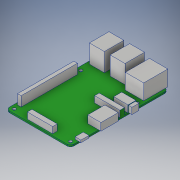
# Autodesk Inventor part: RaspberryPi3B+
Saved by Autodesk Inventor 2017 (Build 210142000, 142)
## iProperties
Created: 2018-08-04
Part Number: RaspberryPi3B+
Material: Aluminum 6061
Document SubType Name: Modeling
Designer: Jake
Density: 2.7 g/cm^3
Appearance: Aluminum - Flat
Author: Jake
Autodesk Inventor part; units mm, degrees
ref_plane "YZ Plane" through (0, 0, 0) normal (1, 0, 0) x (0, 1, 0)
ref_plane "XZ Plane" through (0, 0, 0) normal (0, 1, 0) x (-1, 0, 0)
ref_plane "XY Plane" through (0, 0, 0) normal (0, 0, 1) x (1, 0, 0)
sketch "Sketch1" plane through (0, 0, 0) normal (0, 1, 0) x (-1, 0, 0)
  line L0 (28, 42.5) -> (-28, 42.5)
  line L1 (-28, 42.5) -> (-28, -42.5)
  line L2 (-28, -42.5) -> (28, -42.5)
  line L3 (28, -42.5) -> (28, 42.5)
  point P0 (0, 0)
  point P1 (28, 0)
  point P2 (0, -42.5)
  dimension "d0" = 85
  dimension "d1" = 56
  constraints: 8 end point, 2 midpoint, 2 parallel, 1 horizontal, 1 horizontal alignment, 1 perpendicular, 1 vertical alignment
  measures "d0" distance of L2.end L0.start
  measures "d1" distance of L1.end L2.end
extrude "Extrusion1" add sketch "Sketch1" along normal blind 1.43
sketch "Sketch2" plane through (0, 1.43, 0) normal (0, 1, 0) x (1, 0, 0)
  line L0 (-28, -42.5) -> (28, -42.5) projected
  line L1 (28, -42.5) -> (28, 42.5) projected
  line L2 (28, 42.5) -> (-28, 42.5) projected
  line L3 (-28, 42.5) -> (-28, -42.5) projected
  circle A0 centre (-24.5, -39) radius 1.375
  circle A1 centre (-24.5, 19) radius 1.375
  circle A2 centre (24.5, 19) radius 1.375
  circle A3 centre (24.5, -39) radius 1.375
  point P0 (0, 0)
  dimension "d4" = 2.75
  dimension "d5" = 2.75
  dimension "d6" = 2.75
  dimension "d7" = 2.75
  dimension "d8" = 49
  dimension "d9" = 58
  dimension "d10" = 3.5
  dimension "d11" = 3.5
  constraints: 4 centre point, 2 horizontal alignment, 2 vertical alignment
  measures "d4" diameter of A0
  measures "d5" diameter of A1
  measures "d6" diameter of A2
  measures "d7" diameter of A3
  measures "d8" distance of A3.centre A0.centre
  measures "d9" distance of A1.centre A0.centre
  measures "d10" distance from line of A3.centre L0
  measures "d11" distance from line of L3 A0.centre
extrude "Extrusion2" cut sketch "Sketch2" against normal through all contours A0 | A1 | A2 | A3
fillet "Fillet1" radius 3 4 edges at (-28, 0.715, 42.5) (28, 0.715, 42.5) (28, 0.715, -42.5) (-28, 0.715, -42.5)
sketch "Sketch3" plane through (0, 1.43, 0) normal (0, 1, 0) x (1, 0, 0)
  circle A0 centre (24.5, 19) radius 1.375 projected
  circle A1 centre (-24.5, -39) radius 1.375 projected
  circle A2 centre (-24.5, 19) radius 1.375 projected
  circle A3 centre (24.5, -39) radius 1.375 projected
  arc A4 (-25, 42.5) -> (-28, 39.5) centre (-25, 39.5) ccw projected
  line L0 (-28, 39.5) -> (-28, -39.5) projected
  arc A5 (-28, -39.5) -> (-25, -42.5) centre (-25, -39.5) ccw projected
  line L1 (-25, -42.5) -> (25, -42.5) projected
  arc A6 (25, -42.5) -> (28, -39.5) centre (25, -39.5) ccw projected
  line L2 (28, -39.5) -> (28, 39.5) projected
  arc A7 (28, 39.5) -> (25, 42.5) centre (25, 39.5) ccw projected
  line L3 (25, 42.5) -> (-25, 42.5) projected
  line L4 (-25.5, 27.5) -> (-12.5, 27.5)
  line L5 (-12.5, 27.5) -> (-12.5, 44.5)
  line L6 (-12.5, 44.5) -> (-25.5, 44.5)
  line L7 (-25.5, 44.5) -> (-25.5, 27.5)
  line L8 (-7.5, 27.5) -> (5.5, 27.5)
  line L9 (5.5, 27.5) -> (5.5, 44.5)
  line L10 (5.5, 44.5) -> (-7.5, 44.5)
  line L11 (-7.5, 44.5) -> (-7.5, 27.5)
  point P0 (0, 0)
  point P1 (-19, 44.5)
  point P2 (-1, 44.5)
  dimension "d15" = 2
  dimension "d16" = 29
  dimension "d17" = 47
  dimension "d18" = 13
  dimension "d19" = 13
  dimension "d20" = 17
  constraints: 16 end point, 4 parallel, 2 horizontal, 2 midpoint, 2 perpendicular, 2 point on line
  measures "d15" distance between parallel lines of L6 L3
  measures "d16" distance from line of point (-1, 44.5) L2
  measures "d17" distance from line of point (-19, 44.5) L2
  measures "d18" distance of L5.end L6.end
  measures "d19" distance of L9.end L10.end
  measures "d20" distance of L6.end L4.start
extrude "Extrusion3" add sketch "Sketch3" along normal blind 16 contours L3 L5 L4 L7 A4 | A4 L7 L6 L5 L3 | L11 L10 L9 L3 | L3 L9 L8 L11
sketch "Sketch4" plane through (0, 1.43, 0) normal (0, 1, 0) x (1, 0, 0)
  line L0 (-7.5, 27.5) -> (-7.5, 42.5) projected
  line L1 (-7.5, 42.5) -> (-12.5, 42.5) projected
  line L2 (-12.5, 42.5) -> (-12.5, 27.5) projected
  line L3 (-12.5, 27.5) -> (-25.5, 27.5) projected
  line L4 (-25.5, 27.5) -> (-25.5, 42.458) projected
  arc A0 (-25.5, 42.458) -> (-28, 39.5) centre (-25, 39.5) ccw projected
  line L5 (-28, 39.5) -> (-28, -39.5) projected
  arc A1 (-28, -39.5) -> (-25, -42.5) centre (-25, -39.5) ccw projected
  line L6 (-25, -42.5) -> (25, -42.5) projected
  arc A2 (25, -42.5) -> (28, -39.5) centre (25, -39.5) ccw projected
  line L7 (28, -39.5) -> (28, 39.5) projected
  arc A3 (28, 39.5) -> (25, 42.5) centre (25, 39.5) ccw projected
  line L8 (25, 42.5) -> (5.5, 42.5) projected
  line L9 (5.5, 42.5) -> (5.5, 27.5) projected
  line L10 (5.5, 27.5) -> (-7.5, 27.5) projected
  circle A4 centre (24.5, 19) radius 1.375 projected
  circle A5 centre (-24.5, -39) radius 1.375 projected
  circle A6 centre (-24.5, 19) radius 1.375 projected
  circle A7 centre (24.5, -39) radius 1.375 projected
  line L11 (-7.5, 27.5) -> (5.5, 27.5) projected
  line L12 (5.5, 27.5) -> (5.5, 44.5) projected
  line L13 (5.5, 44.5) -> (-7.5, 44.5) projected
  line L14 (-7.5, 44.5) -> (-7.5, 27.5) projected
  line L15 (9.75, 23.5) -> (25.75, 23.5)
  line L16 (25.75, 23.5) -> (25.75, 44.5)
  line L17 (25.75, 44.5) -> (9.75, 44.5)
  line L18 (9.75, 44.5) -> (9.75, 23.5)
  point P0 (0, 0)
  point P1 (17.75, 44.5)
  dimension "d23" = 10.25
  dimension "d24" = 21
  dimension "d25" = 16
  constraints: 8 end point, 2 parallel, 1 collinear, 1 horizontal, 1 midpoint, 1 perpendicular
  measures "d23" distance from line of point (17.75, 44.5) L7
  measures "d24" distance of L17.end L15.start
  measures "d25" distance of L16.end L17.end
extrude "Extrusion4" add sketch "Sketch4" along normal blind 13.5 contours L18 L17 L16 A3 L8 | L8 A3 L16 L15 L18
sketch "Sketch5" plane through (0, 1.43, 0) normal (0, 1, 0) x (1, 0, 0)
  line L0 (9.75, 23.5) -> (9.75, 42.5) projected
  line L1 (9.75, 42.5) -> (5.5, 42.5) projected
  line L2 (5.5, 42.5) -> (5.5, 27.5) projected
  line L3 (5.5, 27.5) -> (-7.5, 27.5) projected
  line L4 (-7.5, 27.5) -> (-7.5, 42.5) projected
  line L5 (-7.5, 42.5) -> (-12.5, 42.5) projected
  line L6 (-12.5, 42.5) -> (-12.5, 27.5) projected
  line L7 (-12.5, 27.5) -> (-25.5, 27.5) projected
  line L8 (-25.5, 27.5) -> (-25.5, 42.458) projected
  arc A0 (-25.5, 42.458) -> (-28, 39.5) centre (-25, 39.5) ccw projected
  line L9 (-28, 39.5) -> (-28, -39.5) projected
  arc A1 (-28, -39.5) -> (-25, -42.5) centre (-25, -39.5) ccw projected
  line L10 (-25, -42.5) -> (25, -42.5) projected
  arc A2 (25, -42.5) -> (28, -39.5) centre (25, -39.5) ccw projected
  line L11 (28, -39.5) -> (28, 39.5) projected
  arc A3 (28, 39.5) -> (25.75, 42.4047) centre (25, 39.5) ccw projected
  line L12 (25.75, 42.4047) -> (25.75, 23.5) projected
  line L13 (25.75, 23.5) -> (9.75, 23.5) projected
  circle A4 centre (24.5, 19) radius 1.375 projected
  circle A5 centre (-24.5, -39) radius 1.375 projected
  circle A6 centre (-24.5, 19) radius 1.375 projected
  circle A7 centre (24.5, -39) radius 1.375 projected
  line L14 (-26.075, -34.5) -> (-22.925, -34.5)
  line L15 (-22.925, -34.5) -> (-22.925, 14.5)
  line L16 (-22.925, 14.5) -> (-26.075, 14.5)
  line L17 (-26.075, 14.5) -> (-26.075, -34.5)
  point P0 (0, 0)
  point P1 (-26.075, -10)
  point P2 (-24.5, -34.5)
  dimension "d28" = 3.15
  dimension "d29" = 49
  dimension "d31" = 29
  constraints: 8 end point, 2 midpoint, 2 parallel, 1 horizontal, 1 perpendicular, 1 vertical alignment
  measures "d28" distance of L15.end L16.end
  measures "d29" distance of L16.end L14.start
  measures "d31" vertical distance of point (-26.075, -10) A5.centre
extrude "Extrusion5" add sketch "Sketch5" along normal blind 8.5 contours L17 L16 L15 L14
sketch "Sketch6" plane through (0, 1.43, 0) normal (0, 1, 0) x (1, 0, 0)
  line L0 (-26.075, -34.5) -> (-26.075, 14.5) projected
  line L1 (-26.075, 14.5) -> (-22.925, 14.5) projected
  line L2 (-22.925, 14.5) -> (-22.925, -34.5) projected
  line L3 (-22.925, -34.5) -> (-26.075, -34.5) projected
  line L4 (9.75, 23.5) -> (9.75, 42.5) projected
  line L5 (9.75, 42.5) -> (5.5, 42.5) projected
  line L6 (5.5, 42.5) -> (5.5, 27.5) projected
  line L7 (5.5, 27.5) -> (-7.5, 27.5) projected
  line L8 (-7.5, 27.5) -> (-7.5, 42.5) projected
  line L9 (-7.5, 42.5) -> (-12.5, 42.5) projected
  line L10 (-12.5, 42.5) -> (-12.5, 27.5) projected
  line L11 (-12.5, 27.5) -> (-25.5, 27.5) projected
  line L12 (-25.5, 27.5) -> (-25.5, 42.458) projected
  arc A0 (-25.5, 42.458) -> (-28, 39.5) centre (-25, 39.5) ccw projected
  line L13 (-28, 39.5) -> (-28, -39.5) projected
  arc A1 (-28, -39.5) -> (-25, -42.5) centre (-25, -39.5) ccw projected
  line L14 (-25, -42.5) -> (25, -42.5) projected
  arc A2 (25, -42.5) -> (28, -39.5) centre (25, -39.5) ccw projected
  line L15 (28, -39.5) -> (28, 39.5) projected
  arc A3 (28, 39.5) -> (25.75, 42.4047) centre (25, 39.5) ccw projected
  line L16 (25.75, 42.4047) -> (25.75, 23.5) projected
  line L17 (25.75, 23.5) -> (9.75, 23.5) projected
  circle A4 centre (24.5, 19) radius 1.375 projected
  circle A5 centre (-24.5, -39) radius 1.375 projected
  circle A6 centre (-24.5, 19) radius 1.375 projected
  circle A7 centre (24.5, -39) radius 1.375 projected
  line L18 (18.5, -18) -> (30, -18)
  line L19 (30, -18) -> (30, -3)
  line L20 (30, -3) -> (18.5, -3)
  line L21 (18.5, -3) -> (18.5, -18)
  point P0 (0, 0)
  point P1 (30, -10.5)
  dimension "d34" = 2
  dimension "d35" = 11.5
  dimension "d36" = 15
  dimension "d37" = 32
  constraints: 8 end point, 2 parallel, 1 horizontal, 1 midpoint, 1 perpendicular
  measures "d34" distance between parallel lines of L15 L19
  measures "d35" distance of L19.end L20.end
  measures "d36" distance of L20.end L18.start
  measures "d37" distance from line of point (30, -10.5) L14
extrude "Extrusion6" add sketch "Sketch6" along normal blind 6.5 contours L20 L19 L18 L15 | L15 L18 L21 L20
sketch "Sketch7" plane through (0, 1.43, 0) normal (0, 1, 0) x (1, 0, 0)
  line L0 (18.5, -3) -> (28, -3) projected
  line L1 (28, -3) -> (28, 39.5) projected
  arc A0 (28, 39.5) -> (25.75, 42.4047) centre (25, 39.5) ccw projected
  line L2 (25.75, 42.4047) -> (25.75, 23.5) projected
  line L3 (25.75, 23.5) -> (9.75, 23.5) projected
  line L4 (9.75, 23.5) -> (9.75, 42.5) projected
  line L5 (9.75, 42.5) -> (5.5, 42.5) projected
  line L6 (5.5, 42.5) -> (5.5, 27.5) projected
  line L7 (5.5, 27.5) -> (-7.5, 27.5) projected
  line L8 (-7.5, 27.5) -> (-7.5, 42.5) projected
  line L9 (-7.5, 42.5) -> (-12.5, 42.5) projected
  line L10 (-12.5, 42.5) -> (-12.5, 27.5) projected
  line L11 (-12.5, 27.5) -> (-25.5, 27.5) projected
  line L12 (-25.5, 27.5) -> (-25.5, 42.458) projected
  arc A1 (-25.5, 42.458) -> (-28, 39.5) centre (-25, 39.5) ccw projected
  line L13 (-28, 39.5) -> (-28, -39.5) projected
  arc A2 (-28, -39.5) -> (-25, -42.5) centre (-25, -39.5) ccw projected
  line L14 (-25, -42.5) -> (25, -42.5) projected
  arc A3 (25, -42.5) -> (28, -39.5) centre (25, -39.5) ccw projected
  line L15 (28, -39.5) -> (28, -18) projected
  line L16 (28, -18) -> (18.5, -18) projected
  line L17 (18.5, -18) -> (18.5, -3) projected
  line L18 (-26.075, -34.5) -> (-26.075, 14.5) projected
  line L19 (-26.075, 14.5) -> (-22.925, 14.5) projected
  line L20 (-22.925, 14.5) -> (-22.925, -34.5) projected
  line L21 (-22.925, -34.5) -> (-26.075, -34.5) projected
  circle A4 centre (24.5, 19) radius 1.375 projected
  circle A5 centre (-24.5, -39) radius 1.375 projected
  circle A6 centre (-24.5, 19) radius 1.375 projected
  circle A7 centre (24.5, -39) radius 1.375 projected
  line L22 (18.5, -18) -> (30, -18) projected
  line L23 (30, -18) -> (30, -3) projected
  line L24 (30, -3) -> (18.5, -3) projected
  line L25 (18.5, -3) -> (18.5, -18) projected
  line L26 (28, -39.5) -> (28, 39.5) projected
  line L27 (6, 0.5) -> (28, 0.5)
  line L28 (28, 0.5) -> (28, 4.5)
  line L29 (28, 4.5) -> (6, 4.5)
  line L30 (6, 4.5) -> (6, 0.5)
  line L31 (-11, -41) -> (11, -41)
  line L32 (11, -41) -> (11, -37)
  line L33 (11, -37) -> (-11, -37)
  line L34 (-11, -37) -> (-11, -41)
  point P0 (0, 0)
  point P1 (28, 2.5)
  point P2 (0, -41)
  point P3 (30, -10.5)
  point P4 (11, -39)
  dimension "d40" = 22
  dimension "d41" = 22
  dimension "d42" = 4
  dimension "d43" = 4
  dimension "d44" = 28
  dimension "d45" = 13
  constraints: 16 end point, 4 midpoint, 4 parallel, 2 horizontal, 2 perpendicular, 1 horizontal alignment, 1 point on line
  measures "d40" distance of L32.end L33.end
  measures "d41" distance of L28.end L29.end
  measures "d42" distance of L33.end L31.start
  measures "d43" distance of L29.end L27.start
  measures "d44" distance from line of point (0, -41) L15
  measures "d45" vertical distance of point (30, -10.5) point (28, 2.5)
extrude "Extrusion7" add sketch "Sketch7" along normal blind 5.5 contours L27 L30 L29 L1 | L34 L33 L32 L31
sketch "Sketch8" plane through (0, 1.43, 0) normal (0, 1, 0) x (1, 0, 0)
  circle A0 centre (24.5, -39) radius 1.375 projected
  circle A1 centre (-24.5, 19) radius 1.375 projected
  circle A2 centre (-24.5, -39) radius 1.375 projected
  circle A3 centre (24.5, 19) radius 1.375 projected
  line L0 (-26.075, -34.5) -> (-26.075, 14.5) projected
  line L1 (-26.075, 14.5) -> (-22.925, 14.5) projected
  line L2 (-22.925, 14.5) -> (-22.925, -34.5) projected
  line L3 (-22.925, -34.5) -> (-26.075, -34.5) projected
  line L4 (28, 0.5) -> (6, 0.5) projected
  line L5 (6, 0.5) -> (6, 4.5) projected
  line L6 (6, 4.5) -> (28, 4.5) projected
  line L7 (28, 4.5) -> (28, 39.5) projected
  arc A4 (28, 39.5) -> (25.75, 42.4047) centre (25, 39.5) ccw projected
  line L8 (25.75, 42.4047) -> (25.75, 23.5) projected
  line L9 (25.75, 23.5) -> (9.75, 23.5) projected
  line L10 (9.75, 23.5) -> (9.75, 42.5) projected
  line L11 (9.75, 42.5) -> (5.5, 42.5) projected
  line L12 (5.5, 42.5) -> (5.5, 27.5) projected
  line L13 (5.5, 27.5) -> (-7.5, 27.5) projected
  line L14 (-7.5, 27.5) -> (-7.5, 42.5) projected
  line L15 (-7.5, 42.5) -> (-12.5, 42.5) projected
  line L16 (-12.5, 42.5) -> (-12.5, 27.5) projected
  line L17 (-12.5, 27.5) -> (-25.5, 27.5) projected
  line L18 (-25.5, 27.5) -> (-25.5, 42.458) projected
  arc A5 (-25.5, 42.458) -> (-28, 39.5) centre (-25, 39.5) ccw projected
  line L19 (-28, 39.5) -> (-28, -39.5) projected
  arc A6 (-28, -39.5) -> (-25, -42.5) centre (-25, -39.5) ccw projected
  line L20 (-25, -42.5) -> (25, -42.5) projected
  arc A7 (25, -42.5) -> (28, -39.5) centre (25, -39.5) ccw projected
  line L21 (28, -39.5) -> (28, -18) projected
  line L22 (28, -18) -> (18.5, -18) projected
  line L23 (18.5, -18) -> (18.5, -3) projected
  line L24 (18.5, -3) -> (28, -3) projected
  line L25 (28, -3) -> (28, 0.5) projected
  line L26 (-11, -41) -> (-11, -37) projected
  line L27 (-11, -37) -> (11, -37) projected
  line L28 (11, -37) -> (11, -41) projected
  line L29 (11, -41) -> (-11, -41) projected
  line L30 (15.6, 7.5) -> (28, 7.5)
  line L31 (28, 7.5) -> (28, 14.5)
  line L32 (28, 14.5) -> (15.6, 14.5)
  line L33 (15.6, 14.5) -> (15.6, 7.5)
  line L34 (28, 8) -> (31, 8)
  line L35 (31, 8) -> (31, 14)
  line L36 (31, 14) -> (28, 14)
  line L37 (28, 14) -> (28, 8)
  point P0 (0, 0)
  point P1 (31, 11)
  point P2 (28, 11)
  point P3 (31, 11)
  dimension "d48" = 7
  dimension "d49" = 6
  dimension "d50" = 12.4
  dimension "d51" = 3
  dimension "d52" = 53.5
  constraints: 16 end point, 4 parallel, 2 horizontal, 2 midpoint, 2 perpendicular, 2 point on line, 1 coincident, 1 horizontal alignment
  measures "d48" distance of L32.end L30.start
  measures "d49" distance of L34.end L35.end
  measures "d50" distance of L31.end L32.end
  measures "d51" distance of L35.end L36.end
  measures "d52" distance from line of point (31, 11) L20
extrude "Extrusion8" add sketch "Sketch8" along normal blind 6 contours L30 L33 L32 L7 | L7 L36 L35 L34
sketch "Sketch9" plane through (0, 7.43, 0) normal (0, 1, 0) x (1, 0, 0)
  line L0 (28, 8) -> (31, 8) projected
  line L1 (31, 8) -> (31, 14) projected
  line L2 (31, 14) -> (28, 14) projected
  line L3 (28, 14) -> (28, 14.5) projected
  line L4 (28, 14.5) -> (15.6, 14.5) projected
  line L5 (15.6, 14.5) -> (15.6, 7.5) projected
  line L6 (15.6, 7.5) -> (28, 7.5) projected
  line L7 (28, 7.5) -> (28, 8) projected
  line L8 (28, 8) -> (31, 8)
  line L9 (31, 8) -> (31, 14)
  line L10 (31, 14) -> (28, 14)
  line L11 (28, 14) -> (28, 8)
  point P0 (0, 0)
  constraints: 8 end point, 2 parallel, 1 horizontal, 1 perpendicular
extrude "Extrusion9" cut sketch "Sketch9" against normal blind 0.5 contours L11 L2 L1 L0
sketch "Sketch10" plane through (0, 1.43, 0) normal (0, 1, 0) x (1, 0, 0)
  line L0 (15.6, 14.5) -> (28, 14.5) projected
  line L1 (28, 14.5) -> (28, 39.5) projected
  arc A0 (28, 39.5) -> (25.75, 42.4047) centre (25, 39.5) ccw projected
  line L2 (25.75, 42.4047) -> (25.75, 23.5) projected
  line L3 (25.75, 23.5) -> (9.75, 23.5) projected
  line L4 (9.75, 23.5) -> (9.75, 42.5) projected
  line L5 (9.75, 42.5) -> (5.5, 42.5) projected
  line L6 (5.5, 42.5) -> (5.5, 27.5) projected
  line L7 (5.5, 27.5) -> (-7.5, 27.5) projected
  line L8 (-7.5, 27.5) -> (-7.5, 42.5) projected
  line L9 (-7.5, 42.5) -> (-12.5, 42.5) projected
  line L10 (-12.5, 42.5) -> (-12.5, 27.5) projected
  line L11 (-12.5, 27.5) -> (-25.5, 27.5) projected
  line L12 (-25.5, 27.5) -> (-25.5, 42.458) projected
  arc A1 (-25.5, 42.458) -> (-28, 39.5) centre (-25, 39.5) ccw projected
  line L13 (-28, 39.5) -> (-28, -39.5) projected
  arc A2 (-28, -39.5) -> (-25, -42.5) centre (-25, -39.5) ccw projected
  line L14 (-25, -42.5) -> (25, -42.5) projected
  arc A3 (25, -42.5) -> (28, -39.5) centre (25, -39.5) ccw projected
  line L15 (28, -39.5) -> (28, -18) projected
  line L16 (28, -18) -> (18.5, -18) projected
  line L17 (18.5, -18) -> (18.5, -3) projected
  line L18 (18.5, -3) -> (28, -3) projected
  line L19 (28, -3) -> (28, 0.5) projected
  line L20 (28, 0.5) -> (6, 0.5) projected
  line L21 (6, 0.5) -> (6, 4.5) projected
  line L22 (6, 4.5) -> (28, 4.5) projected
  line L23 (28, 4.5) -> (28, 7.5) projected
  line L24 (28, 7.5) -> (15.6, 7.5) projected
  line L25 (15.6, 7.5) -> (15.6, 14.5) projected
  circle A4 centre (24.5, -39) radius 1.375 projected
  circle A5 centre (-24.5, 19) radius 1.375 projected
  circle A6 centre (-24.5, -39) radius 1.375 projected
  circle A7 centre (24.5, 19) radius 1.375 projected
  line L26 (-26.075, -34.5) -> (-26.075, 14.5) projected
  line L27 (-26.075, 14.5) -> (-22.925, 14.5) projected
  line L28 (-22.925, 14.5) -> (-22.925, -34.5) projected
  line L29 (-22.925, -34.5) -> (-26.075, -34.5) projected
  line L30 (-11, -41) -> (-11, -37) projected
  line L31 (-11, -37) -> (11, -37) projected
  line L32 (11, -37) -> (11, -41) projected
  line L33 (11, -41) -> (-11, -41) projected
  line L34 (25, -35.4) -> (30, -35.4)
  line L35 (30, -35.4) -> (30, -28.4)
  line L36 (30, -28.4) -> (25, -28.4)
  line L37 (25, -28.4) -> (25, -35.4)
  point P0 (0, 0)
  point P1 (30, -31.9)
  dimension "d57" = 2
  dimension "d58" = 10.6
  dimension "d59" = 5
  dimension "d60" = 7
  constraints: 8 end point, 2 parallel, 1 horizontal, 1 midpoint, 1 perpendicular
  measures "d57" distance from line of point (30, -31.9) L15
  measures "d58" distance from line of point (30, -31.9) L14
  measures "d59" distance of L35.end L36.end
  measures "d60" distance of L36.end L34.start
extrude "Extrusion10" add sketch "Sketch10" along normal blind 2 contours L36 L35 L34 L15 | L15 L34 L37 L36
equation "\"d5\" = d4"
equation "\"d6\" = d4"
equation "\"d7\" = d4"
equation "\"d11\" = d10"
equation "\"d19\" = d18"
equation "\"d41\" = d40"
equation "\"d43\" = d42"
body "Solid1"
